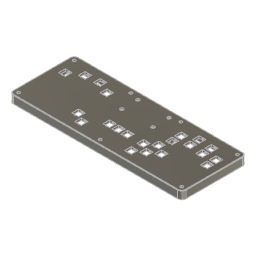
Main Case SH Full (Autodesk Fusion 360 design; units mm, degrees)
Autodesk Fusion 360 part; units mm, degrees
(part 1 of 2)
sketch "Sketch1" plane through (0, 0, 0) normal (0, 0, 1) x (1, 0, 0)
  line L0 (174, -69) -> (-174, -69)
  line L1 (167, 34) -> (153, 34)
  line L2 (141, 31) -> (141, 17)
  line L3 (167, 20) -> (167, 34)
  circle A0 centre (-33, 20) radius 1.6
  line L4 (72, 27) -> (86, 27)
  circle A1 centre (33, 20) radius 1.6
  line L5 (-46, -53) -> (-60, -53)
  line L6 (167, 15) -> (153, 15)
  line L7 (153, 34) -> (153, 20)
  line L8 (153, 20) -> (167, 20)
  line L9 (86, 27) -> (86, 41)
  line L10 (7, -27) -> (-7, -27)
  line L11 (153, 15) -> (153, 1)
  line L12 (-86, 41) -> (-86, 27)
  line L13 (-7, -27) -> (-7, -13)
  circle A2 centre (53, 59) radius 2.6
  arc A3 (174, -69) -> (183, -60) centre (174, -60) ccw
  line L14 (-112, 53) -> (-98, 53)
  line L15 (-65, -40) -> (-65, -26)
  line L16 (127, 50) -> (127, 36)
  line L17 (-127, 36) -> (-127, 50)
  line L18 (-65, -26) -> (-79, -26)
  line L19 (-79, -40) -> (-65, -40)
  line L20 (84, -27) -> (98, -27)
  line L21 (-153, 20) -> (-153, 34)
  arc A4 (-174, 69) -> (-183, 60) centre (-174, 60) ccw
  circle A5 centre (-173, 59) radius 2.6
  line L22 (167, 1) -> (167, 15)
  circle A6 centre (-53, 59) radius 2.6
  line L23 (60, -13) -> (46, -13)
  line L24 (79, -26) -> (65, -26)
  line L25 (-141, 36) -> (-127, 36)
  line L26 (-141, 50) -> (-141, 36)
  line L27 (98, 39) -> (112, 39)
  line L28 (-167, 34) -> (-167, 20)
  line L29 (-7, -13) -> (7, -13)
  line L30 (-174, 69) -> (174, 69)
  line L31 (84, -13) -> (84, -27)
  line L32 (127, 31) -> (141, 31)
  line L33 (112, 39) -> (112, 53)
  line L34 (-60, -53) -> (-60, -39)
  line L35 (112, 53) -> (98, 53)
  line L36 (-98, 39) -> (-112, 39)
  line L37 (98, 20) -> (112, 20)
  line L38 (-72, 27) -> (-72, 41)
  line L39 (112, 34) -> (98, 34)
  line L40 (-72, 41) -> (-86, 41)
  line L41 (141, 36) -> (141, 50)
  line L42 (79, 0) -> (65, 0)
  line L43 (86, 41) -> (72, 41)
  circle A7 centre (-173, -59) radius 2.6
  line L44 (-167, 20) -> (-153, 20)
  line L45 (86, 8) -> (86, 22)
  line L46 (183, 60) -> (183, -60)
  line L47 (112, 20) -> (112, 34)
  line L48 (98, -27) -> (98, -13)
  line L49 (127, 36) -> (141, 36)
  line L50 (-127, 50) -> (-141, 50)
  line L51 (-153, 34) -> (-167, 34)
  line L52 (-183, -60) -> (-183, 60)
  line L53 (46, -13) -> (46, -27)
  line L54 (46, -27) -> (60, -27)
  line L55 (-79, -26) -> (-79, -40)
  circle A8 centre (-33, 54) radius 1.6
  circle A9 centre (33, 54) radius 1.6
  circle A10 centre (173, -59) radius 2.6
  line L56 (60, -27) -> (60, -13)
  line L57 (-46, -39) -> (-46, -53)
  arc A11 (183, 60) -> (174, 69) centre (174, 60) ccw
  line L58 (-112, 39) -> (-112, 53)
  line L59 (65, -26) -> (65, -40)
  line L60 (98, 53) -> (98, 39)
  line L61 (79, -40) -> (79, -26)
  line L62 (-98, 53) -> (-98, 39)
  circle A12 centre (173, 59) radius 2.6
  line L63 (127, 17) -> (127, 31)
  line L64 (72, 8) -> (86, 8)
  line L65 (-86, 27) -> (-72, 27)
  arc A13 (-183, -60) -> (-174, -69) centre (-174, -60) ccw
  line L66 (60, -39) -> (46, -39)
  line L67 (98, -13) -> (84, -13)
  line L68 (141, 50) -> (127, 50)
  line L69 (65, 0) -> (65, -14)
  line L70 (72, 22) -> (72, 8)
  line L71 (98, 34) -> (98, 20)
  line L72 (7, -13) -> (7, -27)
  line L73 (141, 17) -> (127, 17)
  line L74 (65, -14) -> (79, -14)
  line L75 (153, 1) -> (167, 1)
  line L76 (60, -53) -> (60, -39)
  line L77 (46, -53) -> (60, -53)
  line L78 (65, -40) -> (79, -40)
  line L79 (72, 41) -> (72, 27)
  line L80 (86, 22) -> (72, 22)
  line L81 (46, -39) -> (46, -53)
  line L82 (79, -14) -> (79, 0)
  circle A14 centre (0, -59) radius 2.6
  line L83 (-60, -39) -> (-46, -39)
  circle A15 centre (-33, 54) radius 3.5
  circle A16 centre (33, 54) radius 3.5
  circle A17 centre (-33, 20) radius 3.5
  circle A18 centre (33, 20) radius 3.5
  point P0 (91.5, 0)
  point P1 (-91.5, 0)
  dimension "d1" = 9
  dimension "d2" = 3.2
  dimension "d3" = 3.2
  dimension "d4" = 3.2
  dimension "d5" = 3.2
  dimension "d8" = 5.2
  dimension "d9" = 5.2
  dimension "d44" = 7
  dimension "d45" = 7
  dimension "d46" = 7
  dimension "d47" = 7
  constraint horizontal L0
  constraint vertical L46
  constraint vertical L52
  constraint tangent A4 L52
  constraint tangent A4 L30
  constraint tangent L52 A13
  constraint tangent L0 A13
  constraint equal A4 A13
  constraint tangent L0 A3
  constraint tangent A3 L46
  constraint equal A3 A4
  constraint tangent L46 A11
  constraint tangent L30 A11
  constraint equal A4 A11
  constraint concentric A8 A15
  constraint concentric A9 A16
  constraint concentric A0 A17
  constraint concentric A1 A18
  measures "d1" radius of A4
  measures "d2" diameter of A9
  measures "d3" diameter of A1
  measures "d4" diameter of A0
  measures "d5" diameter of A8
  measures "d8" diameter of A6
  measures "d9" diameter of A2
  measures "d44" diameter of A15
  measures "d45" diameter of A16
  measures "d46" diameter of A17
  measures "d47" diameter of A18
extrude "Extrude1" add sketch "Sketch1" against normal blind 4.6 contours L0 A3 A4 L30 L46 L52 A11 A13 | A15 | A16 | A17 | A18
extrude "Extrude6" cut sketch "Sketch1" against normal blind 2.6 contours A15 | A16 | A17 | A18
sketch "Sketch3" plane through (0, 0, -4.6) normal (0, 0, -1) x (1, 0, 0)
  circle A0 centre (33, -20) radius 1.6
  circle A1 centre (-173, -59) radius 2.6
  circle A2 centre (-53, -59) radius 2.6
  line L0 (153, -20) -> (167, -20)
  line L1 (167, -20) -> (167, -34)
  line L2 (167, -34) -> (153, -34)
  line L3 (153, -34) -> (153, -20)
  line L4 (-127, -50) -> (-141, -50)
  line L5 (-141, -50) -> (-141, -36)
  line L6 (-141, -36) -> (-127, -36)
  line L7 (-127, -36) -> (-127, -50)
  circle A3 centre (-173, 59) radius 2.6
  circle A4 centre (53, -59) radius 2.6
  line L8 (-153, -34) -> (-167, -34)
  line L9 (-167, -34) -> (-167, -20)
  line L10 (-167, -20) -> (-153, -20)
  line L11 (-153, -20) -> (-153, -34)
  circle A5 centre (173, 59) radius 2.6
  line L12 (-79, 26) -> (-79, 40)
  line L13 (-79, 40) -> (-65, 40)
  line L14 (-65, 40) -> (-65, 26)
  line L15 (-65, 26) -> (-79, 26)
  circle A6 centre (33, -54) radius 1.6
  circle A7 centre (-33, -54) radius 1.6
  line L16 (60, 27) -> (60, 13)
  line L17 (60, 13) -> (46, 13)
  line L18 (46, 13) -> (46, 27)
  line L19 (46, 27) -> (60, 27)
  line L20 (98, -53) -> (98, -39)
  line L21 (98, -39) -> (112, -39)
  line L22 (112, -39) -> (112, -53)
  line L23 (112, -53) -> (98, -53)
  line L24 (-98, -53) -> (-112, -53)
  line L25 (-112, -53) -> (-112, -39)
  line L26 (-112, -39) -> (-98, -39)
  line L27 (-98, -39) -> (-98, -53)
  line L28 (-86, -27) -> (-72, -27)
  line L29 (-72, -27) -> (-72, -41)
  line L30 (-72, -41) -> (-86, -41)
  line L31 (-86, -41) -> (-86, -27)
  circle A8 centre (173, -59) radius 2.6
  line L32 (98, 13) -> (84, 13)
  line L33 (84, 13) -> (84, 27)
  line L34 (84, 27) -> (98, 27)
  line L35 (98, 27) -> (98, 13)
  line L36 (141, -50) -> (127, -50)
  line L37 (127, -50) -> (127, -36)
  line L38 (127, -36) -> (141, -36)
  line L39 (141, -36) -> (141, -50)
  line L40 (98, -34) -> (98, -20)
  line L41 (98, -20) -> (112, -20)
  line L42 (112, -20) -> (112, -34)
  line L43 (112, -34) -> (98, -34)
  line L44 (7, 13) -> (-7, 13)
  line L45 (-7, 13) -> (-7, 27)
  line L46 (-7, 27) -> (7, 27)
  line L47 (7, 27) -> (7, 13)
  line L48 (141, -17) -> (141, -31)
  line L49 (141, -31) -> (127, -31)
  line L50 (127, -31) -> (127, -17)
  line L51 (127, -17) -> (141, -17)
  line L52 (153, -1) -> (167, -1)
  line L53 (167, -1) -> (167, -15)
  line L54 (167, -15) -> (153, -15)
  line L55 (153, -15) -> (153, -1)
  line L56 (65, 40) -> (79, 40)
  line L57 (79, 40) -> (79, 26)
  line L58 (79, 26) -> (65, 26)
  line L59 (65, 26) -> (65, 40)
  line L60 (72, -41) -> (72, -27)
  line L61 (72, -27) -> (86, -27)
  line L62 (86, -27) -> (86, -41)
  line L63 (86, -41) -> (72, -41)
  line L64 (86, -22) -> (72, -22)
  line L65 (72, -22) -> (72, -8)
  line L66 (72, -8) -> (86, -8)
  line L67 (86, -8) -> (86, -22)
  line L68 (46, 39) -> (46, 53)
  line L69 (46, 53) -> (60, 53)
  line L70 (60, 53) -> (60, 39)
  line L71 (60, 39) -> (46, 39)
  line L72 (79, 14) -> (79, 0)
  line L73 (79, 0) -> (65, 0)
  line L74 (65, 0) -> (65, 14)
  line L75 (65, 14) -> (79, 14)
  line L76 (-60, 39) -> (-60, 53)
  line L77 (-60, 53) -> (-46, 53)
  line L78 (-46, 53) -> (-46, 39)
  line L79 (-46, 39) -> (-60, 39)
  circle A9 centre (0, 59) radius 2.6
  circle A10 centre (-33, -20) radius 1.6
  arc A11 (-183, -60) -> (-174, -69) centre (-174, -60) ccw
  line L80 (-174, -69) -> (174, -69)
  arc A12 (174, -69) -> (183, -60) centre (174, -60) ccw
  line L81 (183, -60) -> (183, 60)
  arc A13 (183, 60) -> (174, 69) centre (174, 60) ccw
  line L82 (174, 69) -> (-174, 69)
  arc A14 (-174, 69) -> (-183, 60) centre (-174, 60) ccw
  line L83 (-183, 60) -> (-183, -60)
  arc A15 (173, -49) -> (163, -59) centre (173, -59) ccw
  arc A16 (163, 59) -> (173, 49) centre (173, 59) ccw
  line L84 (173, 59) -> (170.4, 59)
  line L85 (173, 56.4) -> (173, 59)
  arc A17 (-10, 59) -> (10, 59) centre (0, 59) ccw
  arc A18 (-173, 49) -> (-163, 59) centre (-173, 59) ccw
  arc A19 (-163, -59) -> (-173, -49) centre (-173, -59) ccw
  arc A20 (-43, -59) -> (-63, -59) centre (-53, -59) ccw
  line L86 (-163, -59) -> (-63, -59)
  arc A21 (63, -59) -> (43, -59) centre (53, -59) ccw
  line L87 (-43, -59) -> (43, -59)
  line L88 (63, -59) -> (163, -59)
  line L89 (-173, 49) -> (-173, -49)
  line L90 (-163, 59) -> (-10, 59)
  line L91 (10, 59) -> (163, 59)
  line L92 (173, 49) -> (173, -49)
  circle A22 centre (33, -54) radius 4
  circle A23 centre (33, -20) radius 4
  circle A24 centre (-33, -20) radius 4
  circle A25 centre (-33, -54) radius 4
  circle A26 centre (119.5, 0) radius 12.5
  circle A27 centre (119.5, 0) radius 8.5
  circle A28 centre (-119.5, 0) radius 12.5
  circle A29 centre (-119.5, 0) radius 8.5
  circle A30 centre (-55, -27) radius 12.5
  circle A31 centre (-55, -27) radius 8.5
  circle A32 centre (55, -27) radius 12.5
  circle A33 centre (55, -27) radius 8.5
  point P0 (119.5, 0)
  point P1 (-119.5, 0)
  dimension "d12" = 20
  dimension "d13" = 20
  dimension "d14" = 20
  dimension "d16" = 20
  dimension "d17" = 20
  dimension "d18" = 20
  dimension "d38" = 2.4
  dimension "d39" = 2.4
  dimension "d40" = 2.4
  dimension "d41" = 2.4
  dimension "d253" = 25
  dimension "d254" = -4
  dimension "d255" = 25
  dimension "d256" = -4
  dimension "d259" = 17
  dimension "d260" = 25
  dimension "d261" = -4
  dimension "d262" = 17
  dimension "d263" = 25
  dimension "d264" = -4
  constraint horizontal L86
  constraint parallel L84 L86
  constraint concentric A4 A21
  constraint concentric A2 A20
  constraint concentric A3 A18
  constraint concentric A9 A17
  constraint concentric A5 A16
  constraint coincident A16.start L84
  constraint coincident A5 L84.end
  constraint coincident A5 L85.start
  constraint coincident A20.start L86
  constraint collinear L86 L87
  constraint coincident A21.start L87
  constraint collinear L87 L88
  constraint vertical L89
  constraint horizontal L90
  constraint parallel L84 L91
  constraint vertical L92
  constraint coincident P0 A26.centre
  constraint coincident P1 A28.centre
  measures "d12" diameter of A15
  measures "d13" diameter of A21
  measures "d14" diameter of A20
  measures "d16" diameter of A18
  measures "d17" diameter of A17
  measures "d18" diameter of A16
  measures "d253" diameter of A26
  measures "d255" diameter of A28
  measures "d259" distance of L28.end A30.centre
  measures "d260" diameter of A30
  measures "d262" distance of L60.end A32.centre
  measures "d263" diameter of A32
extrude "Extrude5" add sketch "Sketch3" along normal blind 1.2 contours A22 | A23 | A24 | A25
extrude "Extrude47" add sketch "Sketch3" along normal blind 12 contours A26 | A28 | A30 | A32
extrude "Extrude2" add sketch "Sketch3" along normal blind 12 contours A11 L80 A12 L81 A13 L82 A14 L83
sketch "Sketch4" plane through (0, 0, -16.6) normal (0, 0, -1) x (1, 0, 0)
  circle A0 centre (173, 59) radius 2.6
  circle A1 centre (-173, -59) radius 2.6
  circle A2 centre (173, -59) radius 2.6
  circle A3 centre (53, -59) radius 2.6
  circle A4 centre (-173, 59) radius 2.6
  line L0 (-173, -49) -> (-173, 49)
  arc A5 (-173, 49) -> (-163, 59) centre (-173, 59) ccw
  line L1 (-163, 59) -> (-10, 59)
  arc A6 (-10, 59) -> (10, 59) centre (0, 59) ccw
  line L2 (10, 59) -> (163, 59)
  arc A7 (163, 59) -> (173, 49) centre (173, 59) ccw
  line L3 (173, 49) -> (173, -49)
  arc A8 (173, -49) -> (163, -59) centre (173, -59) ccw
  line L4 (163, -59) -> (63, -59)
  arc A9 (63, -59) -> (43, -59) centre (53, -59) ccw
  line L5 (43, -59) -> (-43, -59)
  arc A10 (-43, -59) -> (-63, -59) centre (-53, -59) ccw
  line L6 (-63, -59) -> (-163, -59)
  arc A11 (-163, -59) -> (-173, -49) centre (-173, -59) ccw
  circle A12 centre (0, 59) radius 2.6
  circle A13 centre (-53, -59) radius 2.6
  line L7 (-183, 60) -> (-183, -60)
  arc A14 (-183, -60) -> (-174, -69) centre (-174, -60) ccw
  line L8 (-174, -69) -> (174, -69)
  arc A15 (174, -69) -> (183, -60) centre (174, -60) ccw
  line L9 (183, -60) -> (183, 60)
  arc A16 (183, 60) -> (174, 69) centre (174, 60) ccw
  line L10 (174, 69) -> (-174, 69)
  arc A17 (-174, 69) -> (-183, 60) centre (-174, 60) ccw
  circle A18 centre (173, -59) radius 3.25
  circle A19 centre (53, -59) radius 3.25
  circle A20 centre (-53, -59) radius 3.25
  circle A21 centre (-173, -59) radius 3.25
  circle A22 centre (-173, 59) radius 3.25
  circle A23 centre (0, 59) radius 3.25
  circle A24 centre (173, 59) radius 3.25
  line L11 (174, -69) -> (16.2321, -69)
  line L12 (163, -59) -> (12.344, -59)
  line L13 (13.3586, -66.862) -> (11.3862, -60.2873)
  line L14 (-174, -69) -> (-16.2321, -69)
  line L15 (-163, -59) -> (-12.344, -59)
  line L16 (-11.3862, -60.2873) -> (-13.3586, -66.862)
  arc A25 (12.344, -59) -> (11.3862, -60.2873) centre (12.344, -60) ccw
  arc A26 (-11.3862, -60.2873) -> (-12.344, -59) centre (-12.344, -60) ccw
  arc A27 (13.3586, -66.862) -> (16.2321, -69) centre (16.2321, -66) ccw
  arc A28 (-16.2321, -69) -> (-13.3586, -66.862) centre (-16.2321, -66) ccw
  point P0 (14, -69)
  point P1 (11, -59)
  point P2 (-14, -69)
  point P3 (-11, -59)
  dimension "d21" = 6.5
  dimension "d22" = 6.5
  dimension "d23" = 6.5
  dimension "d24" = 6.5
  dimension "d25" = 6.5
  dimension "d26" = 6.5
  dimension "d27" = 6.5
  dimension "d30" = 160
  dimension "d31" = 152
  dimension "d32" = 160
  dimension "d33" = 152
  dimension "d34" = 1
  dimension "d35" = 3
  constraint concentric A8 A18
  constraint concentric A3 A19
  constraint concentric A10 A20
  constraint concentric A1 A21
  constraint concentric A4 A22
  constraint concentric A6 A23
  constraint concentric A0 A24
  constraint coincident L8.end A15.start
  constraint parallel L8 L11
  constraint coincident A8.end L4.start
  constraint perpendicular L9 L12
  constraint coincident A14.end L8.start
  constraint parallel L8 L14
  constraint coincident L6.end A11.start
  constraint parallel L6 L15
  constraint coincident P1 L12
  constraint coincident P1 L13
  constraint tangent L12 A25
  constraint tangent L13 A25
  constraint coincident P3 L15
  constraint coincident P3 L16
  constraint tangent L15 A26
  constraint tangent L16 A26
  constraint equal A25 A26
  constraint coincident P0 L11
  constraint coincident P0 L13
  constraint tangent L11 A27
  constraint tangent L13 A27
  constraint coincident P2 L14
  constraint coincident P2 L16
  constraint tangent L14 A28
  constraint tangent L16 A28
  constraint equal A27 A28
  measures "d21" diameter of A18
  measures "d22" diameter of A19
  measures "d23" diameter of A20
  measures "d24" diameter of A21
  measures "d25" diameter of A22
  measures "d26" diameter of A23
  measures "d27" diameter of A24
  measures "d30" distance of L8.end P0
  measures "d31" distance of A8.end P1
  measures "d32" distance of A14.end P2
  measures "d33" distance of L6.end P3
  measures "d34" radius of A25
  measures "d35" radius of A27
extrude "Extrude4" cut sketch "Sketch4" against normal blind 12 contours L5 L8 L13 L16 A25 A26 A27 A28
extrude "Extrude3" cut sketch "Sketch4" against normal blind 6 contours A3 A19 L12 | A3 A19 L12 | A13 A20 L15 | A13 A20 L15 | A18 | A21 | A22 | A23 | A24
sketch "Sketch5" plane through (0, 34, 0) normal (0, -1, 0) x (1, 0, 0)
  line L0 (-153, 0) -> (-167, 0)
  line L1 (-167, 0) -> (-167, -4.6)
  line L2 (-167, -4.6) -> (-153, -4.6)
  line L3 (-153, -4.6) -> (-153, 0)
  line L4 (-160, 0) -> (-160, -2.1)
  line L5 (-158, -2.8) -> (-162, -2.8)
  line L6 (-162, -2.8) -> (-162, -1.4)
  line L7 (-162, -1.4) -> (-158, -1.4)
  line L8 (-158, -1.4) -> (-158, -2.8)
  line L9 (-158, -2.8) -> (-162, -1.4) construction
  line L10 (-162, -2.8) -> (-158, -1.4) construction
  point P0 (-160, -2.1)
  dimension "d50" = 2.1
  dimension "d51" = 4
  dimension "d52" = 1.4
  constraint midpoint L0 L4.start
  constraint perpendicular L0 L4
  constraint horizontal L5
  constraint perpendicular L5 L6
  constraint parallel L5 L7
  constraint parallel L6 L8
  constraint coincident L9 P0
  constraint coincident L10 P0
  constraint coincident P0 L4.end
  measures "d50" distance of L4.start P0
  measures "d51" distance of L6.end L7.end
  measures "d52" distance of L5.end L6.end
extrude "Extrude7" cut sketch "Sketch5" against normal blind 1 contours L5 L6 L7 L8
sketch "Sketch6" plane through (0, 20, 0) normal (0, 1, 0) x (-1, 0, 0)
  line L0 (167, 0) -> (153, 0)
  line L1 (153, 0) -> (153, -4.6)
  line L2 (153, -4.6) -> (167, -4.6)
  line L3 (167, -4.6) -> (167, 0)
  line L4 (160, 0) -> (160, -2.1)
  line L5 (162, -2.8) -> (158, -2.8)
  line L6 (158, -2.8) -> (158, -1.4)
  line L7 (158, -1.4) -> (162, -1.4)
  line L8 (162, -1.4) -> (162, -2.8)
  line L9 (162, -2.8) -> (158, -1.4) construction
  line L10 (158, -2.8) -> (162, -1.4) construction
  point P0 (160, -2.1)
  dimension "d55" = 2.1
  dimension "d56" = 4
  dimension "d57" = 1.4
  constraint midpoint L0 L4.start
  constraint perpendicular L0 L4
  constraint horizontal L5
  constraint perpendicular L5 L6
  constraint parallel L5 L7
  constraint parallel L6 L8
  constraint coincident L9 P0
  constraint coincident L10 P0
  constraint coincident P0 L4.end
  measures "d55" distance of L4.start P0
  measures "d56" distance of L6.end L7.end
  measures "d57" distance of L5.end L6.end
extrude "Extrude8" cut sketch "Sketch6" against normal blind 1 contours L5 L6 L7 L8
sketch "Sketch7" plane through (0, 50, 0) normal (0, -1, 0) x (1, 0, 0)
  line L0 (-127, 0) -> (-141, 0)
  line L1 (-141, 0) -> (-141, -4.6)
  line L2 (-141, -4.6) -> (-127, -4.6)
  line L3 (-127, -4.6) -> (-127, 0)
  line L4 (-134, 0) -> (-134, -2.1)
  line L5 (-132, -1.4) -> (-136, -1.4)
  line L6 (-136, -1.4) -> (-136, -2.8)
  line L7 (-136, -2.8) -> (-132, -2.8)
  line L8 (-132, -2.8) -> (-132, -1.4)
  line L9 (-132, -1.4) -> (-136, -2.8) construction
  line L10 (-136, -1.4) -> (-132, -2.8) construction
  point P0 (-134, -2.1)
  dimension "d60" = 2.1
  dimension "d61" = 4
  dimension "d62" = 1.4
  constraint midpoint L0 L4.start
  constraint perpendicular L0 L4
  constraint horizontal L5
  constraint perpendicular L5 L6
  constraint parallel L5 L7
  constraint parallel L6 L8
  constraint coincident L9 P0
  constraint coincident L10 P0
  constraint coincident P0 L4.end
  measures "d60" distance of L4.start P0
  measures "d61" distance of L6.end L7.end
  measures "d62" distance of L5.end L6.end
extrude "Extrude9" cut sketch "Sketch7" against normal blind 1 contours L5 L6 L7 L8
sketch "Sketch8" plane through (0, 36, 0) normal (0, 1, 0) x (-1, 0, 0)
  line L0 (141, 0) -> (127, 0)
  line L1 (127, 0) -> (127, -4.6)
  line L2 (127, -4.6) -> (141, -4.6)
  line L3 (141, -4.6) -> (141, 0)
  line L4 (134, 0) -> (134, -2.1)
  line L5 (136, -2.8) -> (132, -2.8)
  line L6 (132, -2.8) -> (132, -1.4)
  line L7 (132, -1.4) -> (136, -1.4)
  line L8 (136, -1.4) -> (136, -2.8)
  line L9 (136, -2.8) -> (132, -1.4) construction
  line L10 (132, -2.8) -> (136, -1.4) construction
  point P0 (134, -2.1)
  dimension "d65" = 2.1
  dimension "d66" = 4
  dimension "d67" = 1.4
  constraint midpoint L0 L4.start
  constraint perpendicular L0 L4
  constraint horizontal L5
  constraint perpendicular L5 L6
  constraint parallel L5 L7
  constraint parallel L6 L8
  constraint coincident L9 P0
  constraint coincident L10 P0
  constraint coincident P0 L4.end
  measures "d65" distance of L4.start P0
  measures "d66" distance of L6.end L7.end
  measures "d67" distance of L5.end L6.end
extrude "Extrude10" cut sketch "Sketch8" against normal blind 1 contours L5 L6 L7 L8
sketch "Sketch9" plane through (0, 39, 0) normal (0, 1, 0) x (-1, 0, 0)
  line L0 (112, 0) -> (98, 0)
  line L1 (98, 0) -> (98, -4.6)
  line L2 (98, -4.6) -> (112, -4.6)
  line L3 (112, -4.6) -> (112, 0)
  line L4 (105, 0) -> (105, -2.1)
  line L5 (107, -2.8) -> (103, -2.8)
  line L6 (103, -2.8) -> (103, -1.4)
  line L7 (103, -1.4) -> (107, -1.4)
  line L8 (107, -1.4) -> (107, -2.8)
  line L9 (107, -2.8) -> (103, -1.4) construction
  line L10 (103, -2.8) -> (107, -1.4) construction
  point P0 (105, -2.1)
  dimension "d70" = 2.1
  dimension "d71" = 4
  dimension "d72" = 1.4
  constraint midpoint L0 L4.start
  constraint perpendicular L0 L4
  constraint horizontal L5
  constraint perpendicular L5 L6
  constraint parallel L5 L7
  constraint parallel L6 L8
  constraint coincident L9 P0
  constraint coincident L10 P0
  constraint coincident P0 L4.end
  measures "d70" distance of L4.start P0
  measures "d71" distance of L6.end L7.end
  measures "d72" distance of L5.end L6.end
extrude "Extrude11" cut sketch "Sketch9" against normal blind 1 contours L5 L6 L7 L8
sketch "Sketch10" plane through (0, 53, 0) normal (0, -1, 0) x (1, 0, 0)
  line L0 (-98, 0) -> (-112, 0)
  line L1 (-112, 0) -> (-112, -4.6)
  line L2 (-112, -4.6) -> (-98, -4.6)
  line L3 (-98, -4.6) -> (-98, 0)
  line L4 (-105, 0) -> (-105, -2.1)
  line L5 (-103, -2.8) -> (-107, -2.8)
  line L6 (-107, -2.8) -> (-107, -1.4)
  line L7 (-107, -1.4) -> (-103, -1.4)
  line L8 (-103, -1.4) -> (-103, -2.8)
  line L9 (-103, -2.8) -> (-107, -1.4) construction
  line L10 (-107, -2.8) -> (-103, -1.4) construction
  point P0 (-105, -2.1)
  dimension "d75" = 2.1
  dimension "d76" = 4
  dimension "d77" = 1.4
  constraint midpoint L0 L4.start
  constraint perpendicular L0 L4
  constraint horizontal L5
  constraint perpendicular L5 L6
  constraint parallel L5 L7
  constraint parallel L6 L8
  constraint coincident L9 P0
  constraint coincident L10 P0
  constraint coincident P0 L4.end
  measures "d75" distance of L4.start P0
  measures "d76" distance of L6.end L7.end
  measures "d77" distance of L5.end L6.end
extrude "Extrude12" cut sketch "Sketch10" against normal blind 1 contours L5 L6 L7 L8
sketch "Sketch11" plane through (0, 41, 0) normal (0, -1, 0) x (1, 0, 0)
  line L0 (-72, 0) -> (-86, 0)
  line L1 (-86, 0) -> (-86, -4.6)
  line L2 (-86, -4.6) -> (-72, -4.6)
  line L3 (-72, -4.6) -> (-72, 0)
  line L4 (-79, 0) -> (-79, -2.1)
  line L5 (-77, -2.8) -> (-81, -2.8)
  line L6 (-81, -2.8) -> (-81, -1.4)
  line L7 (-81, -1.4) -> (-77, -1.4)
  line L8 (-77, -1.4) -> (-77, -2.8)
  line L9 (-77, -2.8) -> (-81, -1.4) construction
  line L10 (-81, -2.8) -> (-77, -1.4) construction
  point P0 (-79, -2.1)
  dimension "d80" = 2.1
  dimension "d81" = 4
  dimension "d82" = 1.4
  constraint midpoint L0 L4.start
  constraint perpendicular L0 L4
  constraint horizontal L5
  constraint perpendicular L5 L6
  constraint parallel L5 L7
  constraint parallel L6 L8
  constraint coincident L9 P0
  constraint coincident L10 P0
  constraint coincident P0 L4.end
  measures "d80" distance of L4.start P0
  measures "d81" distance of L6.end L7.end
  measures "d82" distance of L5.end L6.end
extrude "Extrude13" cut sketch "Sketch11" against normal blind 1 contours L5 L6 L7 L8
sketch "Sketch12" plane through (0, 27, 0) normal (0, 1, 0) x (-1, 0, 0)
  line L0 (86, 0) -> (72, 0)
  line L1 (72, 0) -> (72, -4.6)
  line L2 (72, -4.6) -> (86, -4.6)
  line L3 (86, -4.6) -> (86, 0)
  line L4 (79, 0) -> (79, -2.1)
  line L5 (81, -2.8) -> (77, -2.8)
  line L6 (77, -2.8) -> (77, -1.4)
  line L7 (77, -1.4) -> (81, -1.4)
  line L8 (81, -1.4) -> (81, -2.8)
  line L9 (81, -2.8) -> (77, -1.4) construction
  line L10 (77, -2.8) -> (81, -1.4) construction
  point P0 (79, -2.1)
  dimension "d85" = 2.1
  dimension "d86" = 4
  dimension "d87" = 1.4
  constraint midpoint L0 L4.start
  constraint perpendicular L0 L4
  constraint horizontal L5
  constraint perpendicular L5 L6
  constraint parallel L5 L7
  constraint parallel L6 L8
  constraint coincident L9 P0
  constraint coincident L10 P0
  constraint coincident P0 L4.end
  measures "d85" distance of L4.start P0
  measures "d86" distance of L6.end L7.end
  measures "d87" distance of L5.end L6.end
extrude "Extrude14" cut sketch "Sketch12" against normal blind 1 contours L5 L6 L7 L8
sketch "Sketch13" plane through (0, -40, 0) normal (0, 1, 0) x (-1, 0, 0)
  line L0 (79, 0) -> (65, 0)
  line L1 (65, 0) -> (65, -4.6)
  line L2 (65, -4.6) -> (79, -4.6)
  line L3 (79, -4.6) -> (79, 0)
  line L4 (72, 0) -> (72, -2.1)
  line L5 (74, -2.8) -> (70, -2.8)
  line L6 (70, -2.8) -> (70, -1.4)
  line L7 (70, -1.4) -> (74, -1.4)
  line L8 (74, -1.4) -> (74, -2.8)
  line L9 (74, -2.8) -> (70, -1.4) construction
  line L10 (70, -2.8) -> (74, -1.4) construction
  point P0 (72, -2.1)
  dimension "d90" = 2.1
  dimension "d91" = 4
  dimension "d92" = 1.4
  constraint midpoint L0 L4.start
  constraint perpendicular L0 L4
  constraint horizontal L5
  constraint perpendicular L5 L6
  constraint parallel L5 L7
  constraint parallel L6 L8
  constraint coincident L9 P0
  constraint coincident L10 P0
  constraint coincident P0 L4.end
  measures "d90" distance of L4.start P0
  measures "d91" distance of L6.end L7.end
  measures "d92" distance of L5.end L6.end
extrude "Extrude15" cut sketch "Sketch13" against normal blind 1 contours L5 L6 L7 L8
sketch "Sketch14" plane through (0, -26, 0) normal (0, -1, 0) x (1, 0, 0)
  line L0 (-65, 0) -> (-79, 0)
  line L1 (-79, 0) -> (-79, -4.6)
  line L2 (-79, -4.6) -> (-65, -4.6)
  line L3 (-65, -4.6) -> (-65, 0)
  line L4 (-72, 0) -> (-72, -2.1)
  line L5 (-70, -2.8) -> (-74, -2.8)
  line L6 (-74, -2.8) -> (-74, -1.4)
  line L7 (-74, -1.4) -> (-70, -1.4)
  line L8 (-70, -1.4) -> (-70, -2.8)
  line L9 (-70, -2.8) -> (-74, -1.4) construction
  line L10 (-74, -2.8) -> (-70, -1.4) construction
  point P0 (-72, -2.1)
  dimension "d95" = 2.1
  dimension "d96" = 4
  dimension "d97" = 1.4
  constraint midpoint L0 L4.start
  constraint perpendicular L0 L4
  constraint horizontal L5
  constraint perpendicular L5 L6
  constraint parallel L5 L7
  constraint parallel L6 L8
  constraint coincident L9 P0
  constraint coincident L10 P0
  constraint coincident P0 L4.end
  measures "d95" distance of L4.start P0
  measures "d96" distance of L6.end L7.end
  measures "d97" distance of L5.end L6.end
extrude "Extrude16" cut sketch "Sketch14" against normal blind 1 contours L5 L6 L7 L8
sketch "Sketch15" plane through (0, -39, 0) normal (0, -1, 0) x (1, 0, 0)
  line L0 (-46, 0) -> (-60, 0)
  line L1 (-60, 0) -> (-60, -4.6)
  line L2 (-60, -4.6) -> (-46, -4.6)
  line L3 (-46, -4.6) -> (-46, 0)
  line L4 (-53, 0) -> (-53, -2.1)
  line L5 (-51, -2.8) -> (-55, -2.8)
  line L6 (-55, -2.8) -> (-55, -1.4)
  line L7 (-55, -1.4) -> (-51, -1.4)
  line L8 (-51, -1.4) -> (-51, -2.8)
  line L9 (-51, -2.8) -> (-55, -1.4) construction
  line L10 (-55, -2.8) -> (-51, -1.4) construction
  point P0 (-53, -2.1)
  dimension "d100" = 2.1
  dimension "d101" = 4
  dimension "d102" = 1.4
  constraint midpoint L0 L4.start
  constraint perpendicular L0 L4
  constraint horizontal L5
  constraint perpendicular L5 L6
  constraint parallel L5 L7
  constraint parallel L6 L8
  constraint coincident L9 P0
  constraint coincident L10 P0
  constraint coincident P0 L4.end
  measures "d100" distance of L4.start P0
  measures "d101" distance of L6.end L7.end
  measures "d102" distance of L5.end L6.end
extrude "Extrude17" cut sketch "Sketch15" against normal blind 1 contours L5 L6 L7 L8
sketch "Sketch16" plane through (0, -53, 0) normal (0, 1, 0) x (-1, 0, 0)
  line L0 (60, 0) -> (46, 0)
  line L1 (46, 0) -> (46, -4.6)
  line L2 (46, -4.6) -> (60, -4.6)
  line L3 (60, -4.6) -> (60, 0)
  line L4 (53, 0) -> (53, -2.1)
  line L5 (55, -2.8) -> (51, -2.8)
  line L6 (51, -2.8) -> (51, -1.4)
  line L7 (51, -1.4) -> (55, -1.4)
  line L8 (55, -1.4) -> (55, -2.8)
  line L9 (55, -2.8) -> (51, -1.4) construction
  line L10 (51, -2.8) -> (55, -1.4) construction
  point P0 (53, -2.1)
  dimension "d105" = 2.1
  dimension "d106" = 4
  dimension "d107" = 1.4
  constraint midpoint L0 L4.start
  constraint perpendicular L0 L4
  constraint horizontal L5
  constraint perpendicular L5 L6
  constraint parallel L5 L7
  constraint parallel L6 L8
  constraint coincident L9 P0
  constraint coincident L10 P0
  constraint coincident P0 L4.end
  measures "d105" distance of L4.start P0
  measures "d106" distance of L6.end L7.end
  measures "d107" distance of L5.end L6.end
extrude "Extrude18" cut sketch "Sketch16" against normal blind 1 contours L5 L6 L7 L8
sketch "Sketch17" plane through (0, -13, 0) normal (0, -1, 0) x (1, 0, 0)
  line L0 (7, 0) -> (-7, 0)
  line L1 (-7, 0) -> (-7, -4.6)
  line L2 (-7, -4.6) -> (7, -4.6)
  line L3 (7, -4.6) -> (7, 0)
  line L4 (0, 0) -> (0, -2.1)
  line L5 (2, -2.8) -> (-2, -2.8)
  line L6 (-2, -2.8) -> (-2, -1.4)
  line L7 (-2, -1.4) -> (2, -1.4)
  line L8 (2, -1.4) -> (2, -2.8)
  line L9 (2, -2.8) -> (-2, -1.4) construction
  line L10 (-2, -2.8) -> (2, -1.4) construction
  point P0 (0, -2.1)
  dimension "d110" = 2.1
  dimension "d111" = 4
  dimension "d112" = 1.4
  constraint coincident L4.start origin
  constraint perpendicular L0 L4
  constraint horizontal L5
  constraint perpendicular L5 L6
  constraint parallel L5 L7
  constraint parallel L6 L8
  constraint coincident L9 P0
  constraint coincident L10 P0
  constraint coincident P0 L4.end
  measures "d110" distance of L4.start P0
  measures "d111" distance of L6.end L7.end
  measures "d112" distance of L5.end L6.end
extrude "Extrude19" cut sketch "Sketch17" against normal blind 1 contours L5 L6 L7 L8
sketch "Sketch18" plane through (0, -27, 0) normal (0, 1, 0) x (-1, 0, 0)
  line L0 (7, 0) -> (-7, 0)
  line L1 (-7, 0) -> (-7, -4.6)
  line L2 (-7, -4.6) -> (7, -4.6)
  line L3 (7, -4.6) -> (7, 0)
  line L4 (0, 0) -> (0, -2.1)
  line L5 (2, -2.8) -> (-2, -2.8)
  line L6 (-2, -2.8) -> (-2, -1.4)
  line L7 (-2, -1.4) -> (2, -1.4)
  line L8 (2, -1.4) -> (2, -2.8)
  line L9 (2, -2.8) -> (-2, -1.4) construction
  line L10 (-2, -2.8) -> (2, -1.4) construction
  point P0 (0, -2.1)
  dimension "d115" = 2.1
  dimension "d116" = 4
  dimension "d117" = 1.4
  constraint coincident L4.start origin
  constraint perpendicular L0 L4
  constraint horizontal L5
  constraint perpendicular L5 L6
  constraint parallel L5 L7
  constraint parallel L6 L8
  constraint coincident L9 P0
  constraint coincident L10 P0
  constraint coincident P0 L4.end
  measures "d115" distance of L4.start P0
  measures "d116" distance of L6.end L7.end
  measures "d117" distance of L5.end L6.end
extrude "Extrude20" cut sketch "Sketch18" against normal blind 1 contours L5 L6 L7 L8
sketch "Sketch19" plane through (0, -13, 0) normal (0, -1, 0) x (1, 0, 0)
  line L0 (60, 0) -> (46, 0)
  line L1 (46, 0) -> (46, -4.6)
  line L2 (46, -4.6) -> (60, -4.6)
  line L3 (60, -4.6) -> (60, 0)
  line L4 (53, 0) -> (53, -2.1)
  line L5 (55, -2.8) -> (51, -2.8)
  line L6 (51, -2.8) -> (51, -1.4)
  line L7 (51, -1.4) -> (55, -1.4)
  line L8 (55, -1.4) -> (55, -2.8)
  line L9 (55, -2.8) -> (51, -1.4) construction
  line L10 (51, -2.8) -> (55, -1.4) construction
  point P0 (53, -2.1)
  dimension "d120" = 2.1
  dimension "d121" = 4
  dimension "d122" = 1.4
  constraint midpoint L0 L4.start
  constraint perpendicular L0 L4
  constraint horizontal L5
  constraint perpendicular L5 L6
  constraint parallel L5 L7
  constraint parallel L6 L8
  constraint coincident L9 P0
  constraint coincident L10 P0
  constraint coincident P0 L4.end
  measures "d120" distance of L4.start P0
  measures "d121" distance of L6.end L7.end
  measures "d122" distance of L5.end L6.end
extrude "Extrude21" cut sketch "Sketch19" against normal blind 1 contours L5 L6 L7 L8
sketch "Sketch20" plane through (0, -27, 0) normal (0, 1, 0) x (-1, 0, 0)
  line L0 (-46, 0) -> (-60, 0)
  line L1 (-60, 0) -> (-60, -4.6)
  line L2 (-60, -4.6) -> (-46, -4.6)
  line L3 (-46, -4.6) -> (-46, 0)
  line L4 (-53, 0) -> (-53, -2.1)
  line L5 (-51, -2.8) -> (-55, -2.8)
  line L6 (-55, -2.8) -> (-55, -1.4)
  line L7 (-55, -1.4) -> (-51, -1.4)
  line L8 (-51, -1.4) -> (-51, -2.8)
  line L9 (-51, -2.8) -> (-55, -1.4) construction
  line L10 (-55, -2.8) -> (-51, -1.4) construction
  point P0 (-53, -2.1)
  dimension "d125" = 2.1
  dimension "d126" = 4
  dimension "d127" = 1.4
  constraint midpoint L0 L4.start
  constraint perpendicular L0 L4
  constraint horizontal L5
  constraint perpendicular L5 L6
  constraint parallel L5 L7
  constraint parallel L6 L8
  constraint coincident L9 P0
  constraint coincident L10 P0
  constraint coincident P0 L4.end
  measures "d125" distance of L4.start P0
  measures "d126" distance of L6.end L7.end
  measures "d127" distance of L5.end L6.end
extrude "Extrude22" cut sketch "Sketch20" against normal blind 1 contours L5 L6 L7 L8
sketch "Sketch21" plane through (0, -53, 0) normal (0, 1, 0) x (-1, 0, 0)
  line L0 (-46, 0) -> (-60, 0)
  line L1 (-60, 0) -> (-60, -4.6)
  line L2 (-60, -4.6) -> (-46, -4.6)
  line L3 (-46, -4.6) -> (-46, 0)
  line L4 (-53, 0) -> (-53, -2.1)
  line L5 (-51, -2.8) -> (-55, -2.8)
  line L6 (-55, -2.8) -> (-55, -1.4)
  line L7 (-55, -1.4) -> (-51, -1.4)
  line L8 (-51, -1.4) -> (-51, -2.8)
  line L9 (-51, -2.8) -> (-55, -1.4) construction
  line L10 (-55, -2.8) -> (-51, -1.4) construction
  point P0 (-53, -2.1)
  dimension "d130" = 2.1
  dimension "d131" = 4
  dimension "d132" = 1.4
  constraint midpoint L0 L4.start
  constraint perpendicular L0 L4
  constraint horizontal L5
  constraint perpendicular L5 L6
  constraint parallel L5 L7
  constraint parallel L6 L8
  constraint coincident L9 P0
  constraint coincident L10 P0
  constraint coincident P0 L4.end
  measures "d130" distance of L4.start P0
  measures "d131" distance of L6.end L7.end
  measures "d132" distance of L5.end L6.end
extrude "Extrude23" cut sketch "Sketch21" against normal blind 1 contours L5 L6 L7 L8
sketch "Sketch22" plane through (0, -39, 0) normal (0, -1, 0) x (1, 0, 0)
  line L0 (60, 0) -> (46, 0)
  line L1 (46, 0) -> (46, -4.6)
  line L2 (46, -4.6) -> (60, -4.6)
  line L3 (60, -4.6) -> (60, 0)
  line L4 (53, 0) -> (53, -2.1)
  line L5 (55, -2.8) -> (51, -2.8)
  line L6 (51, -2.8) -> (51, -1.4)
  line L7 (51, -1.4) -> (55, -1.4)
  line L8 (55, -1.4) -> (55, -2.8)
  line L9 (55, -2.8) -> (51, -1.4) construction
  line L10 (51, -2.8) -> (55, -1.4) construction
  point P0 (53, -2.1)
  dimension "d135" = 2.1
  dimension "d136" = 4
  dimension "d137" = 1.4
  constraint midpoint L0 L4.start
  constraint perpendicular L0 L4
  constraint horizontal L5
  constraint perpendicular L5 L6
  constraint parallel L5 L7
  constraint parallel L6 L8
  constraint coincident L9 P0
  constraint coincident L10 P0
  constraint coincident P0 L4.end
  measures "d135" distance of L4.start P0
  measures "d136" distance of L6.end L7.end
  measures "d137" distance of L5.end L6.end
extrude "Extrude24" cut sketch "Sketch22" against normal blind 1 contours L5 L6 L7 L8
sketch "Sketch23" plane through (0, 0, 0) normal (0, -1, 0) x (1, 0, 0)
  line L0 (79, 0) -> (65, 0)
  line L1 (65, 0) -> (65, -4.6)
  line L2 (65, -4.6) -> (79, -4.6)
  line L3 (79, -4.6) -> (79, 0)
  line L4 (72, 0) -> (72, -2.1)
  line L5 (74, -2.8) -> (70, -2.8)
  line L6 (70, -2.8) -> (70, -1.4)
  line L7 (70, -1.4) -> (74, -1.4)
  line L8 (74, -1.4) -> (74, -2.8)
  line L9 (74, -2.8) -> (70, -1.4) construction
  line L10 (70, -2.8) -> (74, -1.4) construction
  point P0 (72, -2.1)
  dimension "d140" = 2.1
  dimension "d141" = 4
  dimension "d142" = 1.4
  constraint midpoint L0 L4.start
  constraint perpendicular L0 L4
  constraint horizontal L5
  constraint perpendicular L5 L6
  constraint parallel L5 L7
  constraint parallel L6 L8
  constraint coincident L9 P0
  constraint coincident L10 P0
  constraint coincident P0 L4.end
  measures "d140" distance of L4.start P0
  measures "d141" distance of L6.end L7.end
  measures "d142" distance of L5.end L6.end
extrude "Extrude25" cut sketch "Sketch23" against normal blind 1 contours L5 L6 L7 L8
sketch "Sketch24" plane through (0, -14, 0) normal (0, 1, 0) x (-1, 0, 0)
  line L0 (-65, 0) -> (-79, 0)
  line L1 (-79, 0) -> (-79, -4.6)
  line L2 (-79, -4.6) -> (-65, -4.6)
  line L3 (-65, -4.6) -> (-65, 0)
  line L4 (-72, 0) -> (-72, -2.1)
  line L5 (-70, -2.8) -> (-74, -2.8)
  line L6 (-74, -2.8) -> (-74, -1.4)
  line L7 (-74, -1.4) -> (-70, -1.4)
  line L8 (-70, -1.4) -> (-70, -2.8)
  line L9 (-70, -2.8) -> (-74, -1.4) construction
  line L10 (-74, -2.8) -> (-70, -1.4) construction
  point P0 (-72, -2.1)
  dimension "d145" = 2.1
  dimension "d146" = 4
  dimension "d147" = 1.4
  constraint midpoint L0 L4.start
  constraint perpendicular L0 L4
  constraint horizontal L5
  constraint perpendicular L5 L6
  constraint parallel L5 L7
  constraint parallel L6 L8
  constraint coincident L9 P0
  constraint coincident L10 P0
  constraint coincident P0 L4.end
  measures "d145" distance of L4.start P0
  measures "d146" distance of L6.end L7.end
  measures "d147" distance of L5.end L6.end
extrude "Extrude26" cut sketch "Sketch24" against normal blind 1 contours L5 L6 L7 L8
sketch "Sketch25" plane through (0, -40, 0) normal (0, 1, 0) x (-1, 0, 0)
  line L0 (-65, 0) -> (-79, 0)
  line L1 (-79, 0) -> (-79, -4.6)
  line L2 (-79, -4.6) -> (-65, -4.6)
  line L3 (-65, -4.6) -> (-65, 0)
  line L4 (-72, 0) -> (-72, -2.1)
  line L5 (-70, -2.8) -> (-74, -2.8)
  line L6 (-74, -2.8) -> (-74, -1.4)
  line L7 (-74, -1.4) -> (-70, -1.4)
  line L8 (-70, -1.4) -> (-70, -2.8)
  line L9 (-70, -2.8) -> (-74, -1.4) construction
  line L10 (-74, -2.8) -> (-70, -1.4) construction
  point P0 (-72, -2.1)
  dimension "d150" = 2.1
  dimension "d151" = 4
  dimension "d152" = 1.4
  constraint midpoint L0 L4.start
  constraint perpendicular L0 L4
  constraint horizontal L5
  constraint perpendicular L5 L6
  constraint parallel L5 L7
  constraint parallel L6 L8
  constraint coincident L9 P0
  constraint coincident L10 P0
  constraint coincident P0 L4.end
  measures "d150" distance of L4.start P0
  measures "d151" distance of L6.end L7.end
  measures "d152" distance of L5.end L6.end
extrude "Extrude27" cut sketch "Sketch25" against normal blind 1 contours L5 L6 L7 L8
sketch "Sketch26" plane through (0, -26, 0) normal (0, -1, 0) x (1, 0, 0)
  line L0 (79, 0) -> (65, 0)
  line L1 (65, 0) -> (65, -4.6)
  line L2 (65, -4.6) -> (79, -4.6)
  line L3 (79, -4.6) -> (79, 0)
  line L4 (72, 0) -> (72, -2.1)
  line L5 (74, -2.8) -> (70, -2.8)
  line L6 (70, -2.8) -> (70, -1.4)
  line L7 (70, -1.4) -> (74, -1.4)
  line L8 (74, -1.4) -> (74, -2.8)
  line L9 (74, -2.8) -> (70, -1.4) construction
  line L10 (70, -2.8) -> (74, -1.4) construction
  point P0 (72, -2.1)
  dimension "d155" = 2.1
  dimension "d156" = 4
  dimension "d157" = 1.4
  constraint midpoint L0 L4.start
  constraint perpendicular L0 L4
  constraint horizontal L5
  constraint perpendicular L5 L6
  constraint parallel L5 L7
  constraint parallel L6 L8
  constraint coincident L9 P0
  constraint coincident L10 P0
  constraint coincident P0 L4.end
  measures "d155" distance of L4.start P0
  measures "d156" distance of L6.end L7.end
  measures "d157" distance of L5.end L6.end
extrude "Extrude28" cut sketch "Sketch26" against normal blind 1 contours L5 L6 L7 L8
sketch "Sketch27" plane through (0, -13, 0) normal (0, -1, 0) x (1, 0, 0)
  line L0 (98, 0) -> (84, 0)
  line L1 (84, 0) -> (84, -4.6)
  line L2 (84, -4.6) -> (98, -4.6)
  line L3 (98, -4.6) -> (98, 0)
  line L4 (91, 0) -> (91, -2.1)
  line L5 (93, -2.8) -> (89, -2.8)
  line L6 (89, -2.8) -> (89, -1.4)
  line L7 (89, -1.4) -> (93, -1.4)
  line L8 (93, -1.4) -> (93, -2.8)
  line L9 (93, -2.8) -> (89, -1.4) construction
  line L10 (89, -2.8) -> (93, -1.4) construction
  point P0 (91, -2.1)
  dimension "d160" = 2.1
  dimension "d161" = 4
  dimension "d162" = 1.4
  constraint midpoint L0 L4.start
  constraint perpendicular L0 L4
  constraint horizontal L5
  constraint perpendicular L5 L6
  constraint parallel L5 L7
  constraint parallel L6 L8
  constraint coincident L9 P0
  constraint coincident L10 P0
  constraint coincident P0 L4.end
  measures "d160" distance of L4.start P0
  measures "d161" distance of L6.end L7.end
  measures "d162" distance of L5.end L6.end
extrude "Extrude29" cut sketch "Sketch27" against normal blind 1 contours L5 L6 L7 L8
sketch "Sketch28" plane through (0, -27, 0) normal (0, 1, 0) x (-1, 0, 0)
  line L0 (-84, 0) -> (-98, 0)
  line L1 (-98, 0) -> (-98, -4.6)
  line L2 (-98, -4.6) -> (-84, -4.6)
  line L3 (-84, -4.6) -> (-84, 0)
  line L4 (-91, 0) -> (-91, -2.1)
  line L5 (-89, -2.8) -> (-93, -2.8)
  line L6 (-93, -2.8) -> (-93, -1.4)
  line L7 (-93, -1.4) -> (-89, -1.4)
  line L8 (-89, -1.4) -> (-89, -2.8)
  line L9 (-89, -2.8) -> (-93, -1.4) construction
  line L10 (-93, -2.8) -> (-89, -1.4) construction
  point P0 (-91, -2.1)
  dimension "d165" = 2.1
  dimension "d166" = 4
  dimension "d167" = 1.4
  constraint midpoint L0 L4.start
  constraint perpendicular L0 L4
  constraint horizontal L5
  constraint perpendicular L5 L6
  constraint parallel L5 L7
  constraint parallel L6 L8
  constraint coincident L9 P0
  constraint coincident L10 P0
  constraint coincident P0 L4.end
  measures "d165" distance of L4.start P0
  measures "d166" distance of L6.end L7.end
  measures "d167" distance of L5.end L6.end
extrude "Extrude30" cut sketch "Sketch28" against normal blind 1 contours L5 L6 L7 L8
sketch "Sketch29" plane through (0, 22, 0) normal (0, -1, 0) x (1, 0, 0)
  line L0 (86, 0) -> (72, 0)
  line L1 (72, 0) -> (72, -4.6)
  line L2 (72, -4.6) -> (86, -4.6)
  line L3 (86, -4.6) -> (86, 0)
  line L4 (79, 0) -> (79, -2.1)
  line L5 (81, -2.8) -> (77, -2.8)
  line L6 (77, -2.8) -> (77, -1.4)
  line L7 (77, -1.4) -> (81, -1.4)
  line L8 (81, -1.4) -> (81, -2.8)
  line L9 (81, -2.8) -> (77, -1.4) construction
  line L10 (77, -2.8) -> (81, -1.4) construction
  point P0 (79, -2.1)
  dimension "d170" = 2.1
  dimension "d171" = 4
  dimension "d172" = 1.4
  constraint midpoint L0 L4.start
  constraint perpendicular L0 L4
  constraint horizontal L5
  constraint perpendicular L5 L6
  constraint parallel L5 L7
  constraint parallel L6 L8
  constraint coincident L9 P0
  constraint coincident L10 P0
  constraint coincident P0 L4.end
  measures "d170" distance of L4.start P0
  measures "d171" distance of L6.end L7.end
  measures "d172" distance of L5.end L6.end
extrude "Extrude31" cut sketch "Sketch29" against normal blind 1 contours L5 L6 L7 L8
sketch "Sketch30" plane through (0, 8, 0) normal (0, 1, 0) x (-1, 0, 0)
  line L0 (-72, 0) -> (-86, 0)
  line L1 (-86, 0) -> (-86, -4.6)
  line L2 (-86, -4.6) -> (-72, -4.6)
  line L3 (-72, -4.6) -> (-72, 0)
  line L4 (-79, 0) -> (-79, -2.1)
  line L5 (-77, -2.8) -> (-81, -2.8)
  line L6 (-81, -2.8) -> (-81, -1.4)
  line L7 (-81, -1.4) -> (-77, -1.4)
  line L8 (-77, -1.4) -> (-77, -2.8)
  line L9 (-77, -2.8) -> (-81, -1.4) construction
  line L10 (-81, -2.8) -> (-77, -1.4) construction
  point P0 (-79, -2.1)
  dimension "d175" = 2.1
  dimension "d176" = 4
  dimension "d177" = 1.4
  constraint midpoint L0 L4.start
  constraint perpendicular L0 L4
  constraint horizontal L5
  constraint perpendicular L5 L6
  constraint parallel L5 L7
  constraint parallel L6 L8
  constraint coincident L9 P0
  constraint coincident L10 P0
  constraint coincident P0 L4.end
  measures "d175" distance of L4.start P0
  measures "d176" distance of L6.end L7.end
  measures "d177" distance of L5.end L6.end
extrude "Extrude32" cut sketch "Sketch30" against normal blind 1 contours L5 L6 L7 L8
sketch "Sketch31" plane through (0, 27, 0) normal (0, 1, 0) x (-1, 0, 0)
  line L0 (-72, 0) -> (-86, 0)
  line L1 (-86, 0) -> (-86, -4.6)
  line L2 (-86, -4.6) -> (-72, -4.6)
  line L3 (-72, -4.6) -> (-72, 0)
  line L4 (-79, 0) -> (-79, -2.1)
  line L5 (-77, -2.8) -> (-81, -2.8)
  line L6 (-81, -2.8) -> (-81, -1.4)
  line L7 (-81, -1.4) -> (-77, -1.4)
  line L8 (-77, -1.4) -> (-77, -2.8)
  line L9 (-77, -2.8) -> (-81, -1.4) construction
  line L10 (-81, -2.8) -> (-77, -1.4) construction
  point P0 (-79, -2.1)
  dimension "d180" = 2.1
  dimension "d181" = 4
  dimension "d182" = 1.4
  constraint midpoint L0 L4.start
  constraint perpendicular L0 L4
  constraint horizontal L5
  constraint perpendicular L5 L6
  constraint parallel L5 L7
  constraint parallel L6 L8
  constraint coincident L9 P0
  constraint coincident L10 P0
  constraint coincident P0 L4.end
  measures "d180" distance of L4.start P0
  measures "d181" distance of L6.end L7.end
  measures "d182" distance of L5.end L6.end
extrude "Extrude33" cut sketch "Sketch31" against normal blind 1 contours L5 L6 L7 L8
sketch "Sketch32" plane through (0, 41, 0) normal (0, -1, 0) x (1, 0, 0)
  line L0 (86, 0) -> (72, 0)
  line L1 (72, 0) -> (72, -4.6)
  line L2 (72, -4.6) -> (86, -4.6)
  line L3 (86, -4.6) -> (86, 0)
  line L4 (79, 0) -> (79, -2.1)
  line L5 (81, -2.8) -> (77, -2.8)
  line L6 (77, -2.8) -> (77, -1.4)
  line L7 (77, -1.4) -> (81, -1.4)
  line L8 (81, -1.4) -> (81, -2.8)
  line L9 (81, -2.8) -> (77, -1.4) construction
  line L10 (77, -2.8) -> (81, -1.4) construction
  point P0 (79, -2.1)
  dimension "d185" = 2.1
  dimension "d186" = 4
  dimension "d187" = 1.4
  constraint midpoint L0 L4.start
  constraint perpendicular L0 L4
  constraint horizontal L5
  constraint perpendicular L5 L6
  constraint parallel L5 L7
  constraint parallel L6 L8
  constraint coincident L9 P0
  constraint coincident L10 P0
  constraint coincident P0 L4.end
  measures "d185" distance of L4.start P0
  measures "d186" distance of L6.end L7.end
  measures "d187" distance of L5.end L6.end
extrude "Extrude34" cut sketch "Sketch32" against normal blind 1 contours L5 L6 L7 L8
sketch "Sketch33" plane through (0, 0, 0) normal (0, 0, 1) x (1, 0, 0)
sketch "Sketch34" plane through (0, 53, 0) normal (0, -1, 0) x (1, 0, 0)
  line L0 (112, 0) -> (98, 0)
  line L1 (98, 0) -> (98, -4.6)
  line L2 (98, -4.6) -> (112, -4.6)
  line L3 (112, -4.6) -> (112, 0)
  line L4 (105, 0) -> (105, -2.1)
  line L5 (107, -2.8) -> (103, -2.8)
  line L6 (103, -2.8) -> (103, -1.4)
  line L7 (103, -1.4) -> (107, -1.4)
  line L8 (107, -1.4) -> (107, -2.8)
  line L9 (107, -2.8) -> (103, -1.4) construction
  line L10 (103, -2.8) -> (107, -1.4) construction
  point P0 (105, -2.1)
  dimension "d190" = 2.1
  dimension "d191" = 4
  dimension "d192" = 1.4
  constraint midpoint L0 L4.start
  constraint perpendicular L0 L4
  constraint horizontal L5
  constraint perpendicular L5 L6
  constraint parallel L5 L7
  constraint parallel L6 L8
  constraint coincident L9 P0
  constraint coincident L10 P0
  constraint coincident P0 L4.end
  measures "d190" distance of L4.start P0
  measures "d191" distance of L6.end L7.end
  measures "d192" distance of L5.end L6.end
extrude "Extrude35" cut sketch "Sketch34" against normal blind 1 contours L5 L6 L7 L8
sketch "Sketch35" plane through (0, 39, 0) normal (0, 1, 0) x (-1, 0, 0)
  line L0 (-98, 0) -> (-112, 0)
  line L1 (-112, 0) -> (-112, -4.6)
  line L2 (-112, -4.6) -> (-98, -4.6)
  line L3 (-98, -4.6) -> (-98, 0)
  line L4 (-105, 0) -> (-105, -2.1)
  line L5 (-103, -2.8) -> (-107, -2.8)
  line L6 (-107, -2.8) -> (-107, -1.4)
  line L7 (-107, -1.4) -> (-103, -1.4)
  line L8 (-103, -1.4) -> (-103, -2.8)
  line L9 (-103, -2.8) -> (-107, -1.4) construction
  line L10 (-107, -2.8) -> (-103, -1.4) construction
  point P0 (-105, -2.1)
  dimension "d195" = 2.1
  dimension "d196" = 4
  dimension "d197" = 1.4
  constraint midpoint L0 L4.start
  constraint perpendicular L0 L4
  constraint horizontal L5
  constraint perpendicular L5 L6
  constraint parallel L5 L7
  constraint parallel L6 L8
  constraint coincident L9 P0
  constraint coincident L10 P0
  constraint coincident P0 L4.end
  measures "d195" distance of L4.start P0
  measures "d196" distance of L6.end L7.end
  measures "d197" distance of L5.end L6.end
extrude "Extrude36" cut sketch "Sketch35" against normal blind 1 contours L5 L6 L7 L8
sketch "Sketch36" plane through (0, 20, 0) normal (0, 1, 0) x (-1, 0, 0)
  line L0 (-98, 0) -> (-112, 0)
  line L1 (-112, 0) -> (-112, -4.6)
  line L2 (-112, -4.6) -> (-98, -4.6)
  line L3 (-98, -4.6) -> (-98, 0)
  line L4 (-105, 0) -> (-105, -2.1)
  line L5 (-103, -2.8) -> (-107, -2.8)
  line L6 (-107, -2.8) -> (-107, -1.4)
  line L7 (-107, -1.4) -> (-103, -1.4)
  line L8 (-103, -1.4) -> (-103, -2.8)
  line L9 (-103, -2.8) -> (-107, -1.4) construction
  line L10 (-107, -2.8) -> (-103, -1.4) construction
  point P0 (-105, -2.1)
  dimension "d200" = 2.1
  dimension "d201" = 4
  dimension "d202" = 1.4
  constraint midpoint L0 L4.start
  constraint perpendicular L0 L4
  constraint horizontal L5
  constraint perpendicular L5 L6
  constraint parallel L5 L7
  constraint parallel L6 L8
  constraint coincident L9 P0
  constraint coincident L10 P0
  constraint coincident P0 L4.end
  measures "d200" distance of L4.start P0
  measures "d201" distance of L6.end L7.end
  measures "d202" distance of L5.end L6.end
extrude "Extrude37" cut sketch "Sketch36" against normal blind 1 contours L5 L6 L7 L8